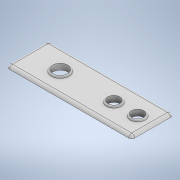
# Autodesk Inventor part: Cover
Saved by Autodesk Inventor 2021 (Build 250183000, 183)
## iProperties
Created: 2021-03-30
Part Number: Cover
Material: Generic
Document SubType Name: Modeling
Designer: eng1-177
Density: 1 g/cm^3
Appearance: Default
Author: eng1-177
Autodesk Inventor part; units mm, degrees
ref_plane "YZ Plane" through (0, 0, 0) normal (1, 0, 0) x (0, 1, 0)
ref_plane "XZ Plane" through (0, 0, 0) normal (0, 1, 0) x (-1, 0, 0)
ref_plane "XY Plane" through (0, 0, 0) normal (0, 0, 1) x (1, 0, 0)
sketch "Sketch1" plane through (0, 0, 0) normal (0, 1, 0) x (-1, 0, 0)
  line L0 (0, 0) -> (-200, 0)
  line L1 (-200, 0) -> (-200, -60)
  line L2 (-200, -60) -> (0, -60)
  line L3 (0, -60) -> (0, 0)
  dimension "d0" = 200
  dimension "d1" = 60
  constraints: 8 end point, 2 parallel, 1 horizontal, 1 perpendicular
  measures "d0" distance of L2.end L1.end
  measures "d1" distance of L1.end L0.end
extrude "Extrusion1" add sketch "Sketch1" along normal blind 2.5
sketch "Sketch2" plane through (0, 0, 0) normal (0, -1, 0) x (1, 0, 0)
  line L0 (200, 0) -> (200, -60) projected
  line L1 (200, 0) -> (180, 0)
  line L2 (180, 0) -> (180, -30)
  line L3 (180, -30) -> (200, -30)
  line L4 (200, -30) -> (200, 0)
  circle A0 centre (180, -30) radius 10
  line L5 (0, 0) -> (200, 0) projected
  line L6 (180, -30) -> (140, -30)
  line L7 (140, -30) -> (140, 0)
  line L8 (140, 0) -> (180, 0)
  line L9 (180, 0) -> (180, -30)
  circle A1 centre (140, -30) radius 10
  dimension "d4" = 20
  dimension "d5" = 30
  dimension "d6" = 20
  dimension "d7" = 40
  constraints: 16 end point, 4 parallel, 2 centre point, 2 coincident, 2 horizontal, 2 perpendicular, 1 point on line
  measures "d4" distance of L3.end L2.end
  measures "d5" distance of L2.end L1.end
  measures "d6" diameter of A0
  measures "d7" distance of L7.end L8.end
sketch "Sketch4" plane through (0, 2.5, 0) normal (0, 1, 0) x (1, 0, 0)
  line L0 (0, 0) -> (200, 0)
  line L1 (200, 0) -> (200, -5)
  line L2 (200, -5) -> (0, -5)
  line L3 (0, -5) -> (0, 0)
  line L4 (0, -5) -> (-5, -5)
  line L5 (-5, -5) -> (-5, 65)
  line L6 (-5, 65) -> (0, 65)
  line L7 (0, 65) -> (0, -5)
  line L8 (0, 60) -> (0, 0) projected
  line L9 (0, 0) -> (200, 0)
  line L10 (200, 0) -> (200, 65)
  line L11 (200, 65) -> (0, 65)
  line L12 (0, 65) -> (0, 0)
  line L13 (200, 65) -> (205, 65)
  line L14 (205, 65) -> (205, -5)
  line L15 (205, -5) -> (200, -5)
  line L16 (200, -5) -> (200, 65)
  dimension "d8" = 200
  dimension "d9" = 5
  dimension "d10" = 5
  dimension "d11" = 70
  dimension "d12" = 5
  constraints: 32 end point, 8 parallel, 4 horizontal, 4 perpendicular
  measures "d8" distance of L1.end L2.end
  measures "d9" distance of L0.end L1.end
  measures "d10" distance of L5.end L6.end
  measures "d11" distance of L4.end L5.end
  measures "d12" distance of L14.end L15.end
extrude "Extrusion2" add sketch "Sketch4" along normal blind 5
extrude "Extrusion3" cut sketch "Sketch2" against normal blind 7.5 contours A0 L6 L3 | L3 L2 A0 | L2 L6 A0 | A1 L6 L7 | L7 L6 A1
fillet "Fillet1" radius 5 4 edges at (205, 5, 5) (205, 5, -65) (-5, 5, -65) (-5, 5, 5)
fillet "Fillet2" radius 5 7 edges at (-3.5355, 7.5, 3.5355) (100, 7.5, 5) (203.5355, 7.5, 3.5355) (205, 7.5, -30) (203.5355, 7.5, -63.5355) (-3.5355, 7.5, -63.5355) (-5, 7.5, -30)
sketch "Sketch5" plane through (0, 0, 0) normal (0, -1, 0) x (1, 0, 0)
  line L0 (0, 0) -> (200, 0) projected
  line L1 (200, -60) -> (0, -60) projected
  line L2 (0, 0) -> (50, 0)
  line L3 (50, 0) -> (50, -60)
  line L4 (50, -60) -> (0, -60)
  line L5 (0, -60) -> (0, 0)
  circle A0 centre (50, -30) radius 12.5
  dimension "d19" = 50
  dimension "d20" = 25
  constraints: 8 end point, 2 parallel, 1 centre point, 1 horizontal, 1 midpoint, 1 perpendicular, 1 point on line
  measures "d19" distance of L3.end L4.end
  measures "d20" diameter of A0
extrude "Extrusion4" cut sketch "Sketch5" against normal blind 7.5 contours A0 L3 | L3 A0
sketch "Sketch6" plane through (0, 7.5, 0) normal (0, 1, 0) x (1, 0, 0)
  circle A0 centre (50, 30) radius 12.5 projected
  circle A1 centre (50, 30) radius 15
  circle A2 centre (140, 30) radius 10 projected
  circle A3 centre (140, 30) radius 12.5
  circle A4 centre (180, 30) radius 10 projected
  circle A5 centre (180, 30) radius 12.5
  point P0 (0, 0)
  dimension "d23" = 30
  dimension "d24" = 25
  constraints: 3 centre point, 3 coincident
  measures "d23" diameter of A1
  measures "d24" diameter of A3
extrude "Extrusion5" add sketch "Sketch6" along normal blind 2.5
fillet "Fillet3" radius 2.5 3 edges at (127.5, 10, -30) (167.5, 10, -30) (35, 10, -30)
body "Solid1"
